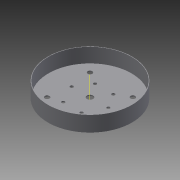
# Autodesk Inventor part: Top Cap
Saved by Autodesk Inventor 2015 (Build 190159000, 159)
## iProperties
Created: 2014-06-24
Part Number: Top Cap
Material: Generic
Document SubType Name: Modeling
Designer: Aki
Density: 1 g/cm^3
Appearance: Default
Author: Aki
Autodesk Inventor part; units mm, degrees
ref_plane "YZ Plane" through (0, 0, 0) normal (1, 0, 0) x (0, 1, 0)
ref_plane "XZ Plane" through (0, 0, 0) normal (0, 1, 0) x (-1, 0, 0)
ref_plane "XY Plane" through (0, 0, 0) normal (0, 0, 1) x (1, 0, 0)
sketch "Sketch1" plane through (0, 0, 0) normal (0, 1, 0) x (-1, 0, 0)
  circle A0 centre (0, 0) radius 87
  circle A1 centre (0, 0) radius 6.35
  circle A2 centre (38.1, 0) radius 3.175
  circle A3 centre (-38.1, 0) radius 3.175
  circle A4 centre (19.05, -29.4637) radius 3.175
  circle A5 centre (-19.05, -29.4637) radius 3.175
  circle A6 centre (19.05, 36.5255) radius 3.175
  circle A7 centre (-19.05, 36.5255) radius 3.175
  circle A8 centre (44.45, -44.45) radius 4.7625
  circle A9 centre (-44.45, -44.45) radius 4.7625
  circle A10 centre (44.45, 44.45) radius 4.7625
  circle A11 centre (-44.45, 44.45) radius 4.7625
  dimension "d1" = 174
  dimension "d7" = 12.7
  dimension "d8" = 6.35
  dimension "d9" = 6.35
  dimension "d10" = 38.1
  dimension "d11" = 38.1
  dimension "d12" = 6.35
  dimension "d13" = 6.35
  dimension "d14" = 6.35
  dimension "d15" = 6.35
  dimension "d16" = 65.9892
  dimension "d17" = 65.9892
  dimension "d18" = 19.05
  dimension "d19" = 19.05
  dimension "d20" = 9.525
  dimension "d21" = 9.525
  dimension "d22" = 9.525
  dimension "d23" = 9.525
  dimension "d24" = 88.9
  dimension "d25" = 88.9
  dimension "d26" = 44.45
  dimension "d27" = 44.45
  dimension "d28" = 88.9
  dimension "d29" = 44.45
  dimension "d30" = 0
  constraints: 12 centre point, 1 coincident
  measures "d1" diameter of A0
  measures "d7" diameter of A1
  measures "d8" diameter of A2
  measures "d9" diameter of A3
  measures "d10" distance of point (0, 0) A2.centre
  measures "d11" distance of A3.centre point (0, 0)
  measures "d12" diameter of A4
  measures "d13" diameter of A5
  measures "d14" diameter of A6
  measures "d15" diameter of A7
  measures "d16" distance of A6.centre A4.centre
  measures "d17" distance of A5.centre A7.centre
  measures "d18" horizontal distance of A4.centre A2.centre
  measures "d19" horizontal distance of A3.centre A5.centre
  measures "d20" diameter of A8
  measures "d21" diameter of A9
  measures "d22" diameter of A10
  measures "d23" diameter of A11
  measures "d24" distance of A11.centre A10.centre
  measures "d25" distance of A9.centre A8.centre
  measures "d26" horizontal distance of A8.centre point (0, 0)
  measures "d27" horizontal distance of point (0, 0) A10.centre
  measures "d28" distance of A8.centre A10.centre
  measures "d29" horizontal distance of A8.centre A0.centre
  measures "d30" distance of point (0, 0) A0.centre
extrude "Extrusion3" add sketch "Sketch1" along normal blind 31.75
sketch "Sketch3" plane through (0, 31.75, 0) normal (0, 1, 0) x (1, 0, 0)
  circle A0 centre (0, 0) radius 86
  dimension "d33" = 172
  constraints: 1 centre point, 1 coincident
  measures "d33" diameter of A0
hole "Hole1" at (0, 31.75, 0) direction (0, -1, 0) diameter 172 depth 29.75
body "Solid2"
